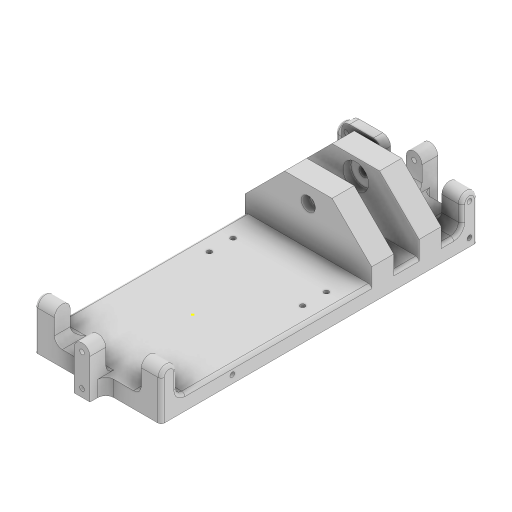
# Autodesk Inventor part: Base
Saved by Autodesk Inventor 2023 (Build 270158000, 158)
## iProperties
Created: 2023-10-18
Part Number: Base
Material: Generic
Document SubType Name: Modeling
Designer: MVeszpremi
Density: 1 g/cm^3
Appearance: Default
Author: MVeszpremi
Autodesk Inventor part; units mm, degrees
ref_plane "YZ Plane" through (0, 0, 0) normal (1, 0, 0) x (0, 1, 0)
ref_plane "XZ Plane" through (0, 0, 0) normal (0, 1, 0) x (-1, 0, 0)
ref_plane "XY Plane" through (0, 0, 0) normal (0, 0, 1) x (1, 0, 0)
sketch "Sketch1" plane through (0, 0, 0) normal (0, 1, 0) x (-1, 0, 0)
  line L0 (40, 60) -> (-40, 60)
  line L1 (-40, 60) -> (-40, -140)
  line L2 (-40, -140) -> (40, -140)
  line L3 (40, -140) -> (40, 60)
  line L4 (29.5, -40) -> (-29.5, -40)
  line L5 (-29.5, -40) -> (-29.5, -55)
  line L6 (-29.5, -55) -> (29.5, -55)
  line L7 (29.5, -55) -> (29.5, -40)
  circle A0 centre (29.5, -40) radius 1.55
  circle A1 centre (29.5, -55) radius 1.55
  circle A2 centre (-29.5, -55) radius 1.55
  circle A3 centre (-29.5, -40) radius 1.55
  point P0 (0, 0)
  dimension "d0" = 40
  dimension "d1" = 80
  dimension "d2" = 59
  dimension "d3" = 15
  dimension "d4" = 29.5
  dimension "d5" = 200
  dimension "d6" = 100
  dimension "d7" = 60
  dimension "d8" = 3.1
  dimension "d9" = 3.1
  dimension "d10" = 3.1
  dimension "d11" = 3.1
  constraints: 16 end point, 4 centre point, 4 coincident, 4 parallel, 2 horizontal, 2 perpendicular
  measures "d0" distance from line of L3 point (0, 0)
  measures "d1" distance of L0.start L0.end
  measures "d2" distance of L4.start L4.end
  measures "d3" distance of L6.end L4.start
  measures "d4" distance from line of point (0, 0) L7
  measures "d5" distance of L2.end L0.start
  measures "d6" distance between parallel lines of L0 L4
  measures "d7" distance from line of L0 point (0, 0)
  measures "d8" diameter of A0
  measures "d9" diameter of A1
  measures "d10" diameter of A3
  measures "d11" diameter of A2
extrude "Extrusion1" add sketch "Sketch1" along normal blind 10 contours L3 L2 L1 L0 | L4 A0 L7 A1 L6 A2 L5 A3
sketch "Sketch2" plane through (0, 0, 0) normal (0, -1, 0) x (1, 0, 0)
  circle A0 centre (29.5, -40) radius 1.55 projected
  line L0 (26.1802, -40) -> (27.8401, -37.125)
  line L1 (27.8401, -37.125) -> (31.1599, -37.125)
  line L2 (31.1599, -37.125) -> (32.8198, -40)
  line L3 (32.8198, -40) -> (31.1599, -42.875)
  line L4 (31.1599, -42.875) -> (27.8401, -42.875)
  line L5 (27.8401, -42.875) -> (26.1802, -40)
  circle A1 centre (29.5, -55) radius 1.55 projected
  line L6 (26.1802, -55) -> (27.8401, -52.125)
  line L7 (27.8401, -52.125) -> (31.1599, -52.125)
  line L8 (31.1599, -52.125) -> (32.8198, -55)
  line L9 (32.8198, -55) -> (31.1599, -57.875)
  line L10 (31.1599, -57.875) -> (27.8401, -57.875)
  line L11 (27.8401, -57.875) -> (26.1802, -55)
  line L12 (0, 0) -> (0, -8.5625)
  circle A2 centre (-29.5, -40) radius 1.55
  line L13 (-26.1802, -40) -> (-27.8401, -37.125)
  line L14 (-27.8401, -37.125) -> (-31.1599, -37.125)
  line L15 (-31.1599, -37.125) -> (-32.8198, -40)
  line L16 (-32.8198, -40) -> (-31.1599, -42.875)
  line L17 (-31.1599, -42.875) -> (-27.8401, -42.875)
  line L18 (-27.8401, -42.875) -> (-26.1802, -40)
  circle A3 centre (-29.5, -55) radius 1.55
  line L19 (-26.1802, -55) -> (-27.8401, -52.125)
  line L20 (-27.8401, -52.125) -> (-31.1599, -52.125)
  line L21 (-31.1599, -52.125) -> (-32.8198, -55)
  line L22 (-32.8198, -55) -> (-31.1599, -57.875)
  line L23 (-31.1599, -57.875) -> (-27.8401, -57.875)
  line L24 (-27.8401, -57.875) -> (-26.1802, -55)
  point P0 (29.5, -42.875)
  point P1 (29.5, -37.125)
  point P2 (-29.5, -42.875)
  point P3 (-29.5, -37.125)
  dimension "d14" = 5.75
  dimension "d15" = 5.75
  constraints: 50 end point, 18 symmetric about line, 4 coincident, 2 centre point, 2 midpoint, 1 vertical, 28 other
  measures "d14" distance of point (29.5, -42.875) point (29.5, -37.125)
  measures "d15" distance between parallel lines of L10 L7
extrude "Extrusion2" cut sketch "Sketch2" against normal blind 3.5 contours A0 | L0 L1 L2 L3 L4 L5 | A1 | L6 L7 L8 L9 L10 L11 | A2 | L18 L17 L16 L15 L14 L13 | A3 | L24 L23 L22 L21 L20 L19
sketch "Sketch3" plane through (0, 10, 0) normal (0, 1, 0) x (1, 0, 0)
  line L0 (-40, 140) -> (-40, -60) projected
  line L1 (40, -60) -> (40, 140) projected
  line L2 (-40, 73.125) -> (40, 73.125)
  line L3 (40, 73.125) -> (40, 87.125)
  line L4 (40, 87.125) -> (-40, 87.125)
  line L5 (-40, 87.125) -> (-40, 73.125)
  circle A0 centre (-29.5, 55) radius 1.55 projected
  line L6 (-40, 140) -> (-40, -60) projected
  line L7 (40, 103.125) -> (-40, 103.125)
  line L8 (-40, 103.125) -> (-40, 117.125)
  line L9 (-40, 117.125) -> (40, 117.125)
  line L10 (40, 117.125) -> (40, 103.125)
  point P0 (0, 0)
  point P1 (-40, 87.125)
  point P2 (40, 73.125)
  point P3 (-40, 117.125)
  point P4 (-40, 103.125)
  dimension "d18" = 18.125
  dimension "d19" = 14
  dimension "d32" = 16
  dimension "d33" = 14
  constraints: 16 end point, 4 parallel, 4 point on line, 2 horizontal, 2 perpendicular
  measures "d18" distance from line of L2 A0.centre
  measures "d19" distance between parallel lines of L4 L2
  measures "d32" distance between parallel lines of L7 L4
  measures "d33" distance between parallel lines of L9 L7
extrude "Extrusion3" add sketch "Sketch3" along normal blind 35 contours L9 L1 L7 L0 | L4 L1 L2 L0
sketch "Sketch4" plane through (40, 10, -87.125) normal (0, 0, -1) x (-1, 0, 0)
  circle A0 centre (40, 24.5) radius 8.125
  line L0 (0, 0) -> (80, 0) projected
  circle A1 centre (40, 24.5) radius 3
  point P0 (40, -10)
  point P1 (40, 0)
  dimension "d22" = 16.25
  dimension "d23" = 24.5
  dimension "d24" = 6
  constraints: 2 centre point, 1 coincident, 1 midpoint
  measures "d22" diameter of A0
  measures "d23" distance of point (40, 0) A0.centre
  measures "d24" diameter of A1
extrude "Extrusion4" cut sketch "Sketch4" along normal blind 40 and the other way blind 20 contours A1
extrude "Extrusion5" cut sketch "Sketch4" along normal blind 21 and the other way blind 5
chamfer "Chamfer1" distance 25 angle 45 4 edges at (40, 45, -80.125) (-40, 45, -80.125) (40, 45, -110.125) (-40, 45, -110.125)
sketch "Sketch5" plane through (-40, 10, -73.125) normal (0, 0, 1) x (1, 0, 0)
  circle A0 centre (40, 24.5) radius 3 projected
  circle A1 centre (40, 24.5) radius 4.5
  point P0 (40, -10)
  dimension "d38" = 9
  constraints: 1 centre point, 1 coincident
  measures "d38" diameter of A1
extrude "Extrusion6" cut sketch "Sketch5" against normal blind 5
ref_plane "Work Plane1" through (-40, 10, -110.125) normal (0, 0, 1) x (1, 0, 0)
mirror "Mirror1" about plane through (-40, 10, -110.125) normal (0, 0, 1) of "Extrusion5"
sketch "Sketch6" plane through (-40, 0, -140) normal (-1, 0, 0) x (0, 0, 1)
  point P0 (140, 0)
sketch "Sketch7" plane through (-40, 0, -140) normal (-1, 0, 0) x (0, 0, 1)
  line L0 (0, 0) -> (0, 10) projected
  line L1 (0, 10) -> (10, 10)
  line L2 (10, 10) -> (10, 30)
  line L3 (10, 30) -> (0, 30)
  line L4 (0, 30) -> (0, 10)
  line L5 (200, 10) -> (66.875, 10) projected
  line L6 (200, 10) -> (190, 10)
  line L7 (190, 10) -> (190, 30)
  line L8 (190, 30) -> (200, 30)
  line L9 (200, 30) -> (200, 10)
  circle A0 centre (5, 25) radius 1.5
  circle A1 centre (155, 25) radius 1.5
  point P0 (140, 0)
  point P1 (190, 10)
  dimension "d41" = 150
  dimension "d42" = 5
  dimension "d43" = 20
  dimension "d44" = 10
  dimension "d45" = 3
  dimension "d46" = 10
  dimension "d47" = 20
  dimension "d48" = 3
  dimension "d51" = 15
  dimension "d52" = 15
  constraints: 16 end point, 4 parallel, 2 centre point, 2 horizontal, 2 perpendicular
  measures "d41" distance of A1.centre A0.centre
  measures "d42" distance from line of L0 A0.centre
  measures "d43" distance of L6.end L7.end
  measures "d44" distance of L7.end L8.end
  measures "d45" diameter of A1
  measures "d46" distance of L2.end L3.end
  measures "d47" distance of L1.end L2.end
  measures "d48" diameter of A0
  measures "d51" distance from line of L5 A1.centre
  measures "d52" distance from line of L1 A0.centre
extrude "Extrusion7" add sketch "Sketch7" against normal blind 12.5 contours L4 L3 L2 L1 | L5 L7 L8 L9
ref_plane "Work Plane2" through (0, 0, -140) normal (-1, 0, 0) x (0, 0, 1)
mirror "Mirror2" about plane through (0, 0, -140) normal (-1, 0, 0) of "Extrusion7"
sketch "Sketch8" plane through (-40, 0, -140) normal (-1, 0, 0) x (0, 0, 1)
  circle A0 centre (5, 5) radius 1.5
  circle A1 centre (155, 5) radius 1.5
  line L0 (0, 0) -> (0, 30) projected
  line L1 (0, 0) -> (200, 0) projected
  point P0 (140, 0)
  dimension "d53" = 150
  dimension "d54" = 5
  dimension "d55" = 5
  dimension "d56" = 3
  dimension "d57" = 3
  constraints: 2 centre point, 1 horizontal alignment
  measures "d53" distance of A1.centre A0.centre
  measures "d54" distance from line of L0 A0.centre
  measures "d55" distance from line of L1 A0.centre
  measures "d56" diameter of A0
  measures "d57" diameter of A1
extrude "Extrusion8" cut sketch "Sketch8" against normal blind 15
mirror "Mirror3" about plane through (0, 0, -140) normal (-1, 0, 0) of "Extrusion8"
sketch "Sketch9" plane through (-40, 0, 60) normal (0, 0, 1) x (1, 0, 0)
  line L0 (0, 0) -> (80, 0) projected
  line L1 (35, 0) -> (45, 0)
  line L2 (45, 0) -> (45, 30)
  line L3 (45, 30) -> (35, 30)
  line L4 (35, 30) -> (35, 0)
  circle A0 centre (40, 25) radius 1.5
  circle A1 centre (40, 5) radius 1.5
  point P0 (40, 0)
  point P1 (40, 0)
  point P2 (40, 0)
  point P3 (40, 0)
  dimension "d60" = 5
  dimension "d61" = 5
  dimension "d62" = 30
  dimension "d63" = 5
  dimension "d64" = 20
  dimension "d65" = 3
  dimension "d66" = 3
  constraints: 8 end point, 3 midpoint, 2 centre point, 2 parallel, 1 horizontal, 1 perpendicular, 1 point on line
  measures "d60" distance from line of L4 point (40, 0)
  measures "d61" distance from line of point (40, 0) L2
  measures "d62" distance of L1.end L2.end
  measures "d63" distance of point (40, 0) A1.centre
  measures "d64" distance of A1.centre A0.centre
  measures "d65" diameter of A0
  measures "d66" diameter of A1
extrude "Extrusion9" add sketch "Sketch9" along normal blind 10
ref_plane "Work Plane3" through (40, 0, -40) normal (0, 0, -1) x (-1, 0, 0)
mirror "Mirror4" about plane through (40, 0, -40) normal (0, 0, -1) of "Extrusion9"
fillet "Fillet1" radius 5 26 edges at (5, 5, 60) (-5, 5, 60) (-5, 30, 65) (5, 30, 65) (-33.75, 30, 60) (-33.75, 30, 50) (33.75, 30, 60) (33.75, 30, 50) (27.5, 10, 55) (-27.5, 10, 55) (33.75, 10, 50) (-33.75, 10, 50) (33.75, 30, -140) (33.75, 30, -130) (33.75, 10, -130) (5, 30, -145) (-5, 30, -145) (0, 10, -140) (0, 10, 60) (-5, 5, -140) (5, 5, -140) (-27.5, 10, -135) (-33.75, 30, -140) (-33.75, 30, -130) (-33.75, 10, -130) (27.5, 10, -135)
fillet "Fillet2" radius 2 22 edges at (-40, 11.4645, 48.5355) (-40, 20, 50) (-40, 30, 55) (-40, 12.5, 60) (-40, 10, -14.0625) (-40, 10, -95.125) (-40, 11.4645, -128.5355) (-40, 20, -130) (-40, 30, -135) (-40, 12.5, -140) (-40, 10, -121.0625) (40, 11.4645, 48.5355) (40, 20, 50) (40, 30, 55) (40, 12.5, 60) (40, 10, -14.0625) (40, 10, -95.125) (40, 11.4645, -128.5355) (40, 20, -130) (40, 30, -135) (40, 12.5, -140) (40, 10, -121.0625)
sketch "Sketch10" plane through (0, 10, 0) normal (0, 1, 0) x (1, 0, 0)
  point P0 (0, 0)
sketch "Sketch11" plane through (0, 10, 0) normal (0, 1, 0) x (1, 0, 0)
  line L0 (-5, 124.125) -> (-30, 124.125)
  line L1 (-30, 124.125) -> (-30, 130.125)
  line L2 (-30, 130.125) -> (-5, 130.125)
  line L3 (-5, 130.125) -> (-5, 124.125)
  line L4 (15, 117.125) -> (-15, 117.125) projected
  point P0 (0, 0)
  dimension "d71" = 5
  dimension "d72" = 25
  dimension "d73" = 6
  dimension "d76" = 7
  constraints: 8 end point, 2 parallel, 1 horizontal, 1 perpendicular
  measures "d71" horizontal distance of L2.end point (0, 0)
  measures "d72" distance of L0.start L0.end
  measures "d73" distance of L0.end L1.end
  measures "d76" distance between parallel lines of L4 L0
extrude "Extrusion10" add sketch "Sketch11" along normal blind 30
sketch "Sketch12" plane through (-5, 10, -130.125) normal (0, 0, -1) x (-1, 0, 0)
  circle A0 centre (3, 24.5) radius 1.5
  circle A1 centre (22, 24.5) radius 1.5
  line L0 (0, 30) -> (25, 30) projected
  line L1 (12.5, 30) -> (12.5, 24.5)
  circle A2 centre (-5, 24.5) radius 3 projected
  line L2 (8.5, 28) -> (16.5, 28)
  line L3 (16.5, 28) -> (16.5, 21)
  line L4 (16.5, 21) -> (8.5, 21)
  line L5 (8.5, 21) -> (8.5, 28)
  point P0 (-5, -10)
  point P1 (12.5, 27.25)
  dimension "d77" = 3
  dimension "d78" = 3
  dimension "d79" = 9.5
  dimension "d80" = 9.5
  dimension "d81" = 7
  dimension "d82" = 2
  dimension "d83" = 8
  dimension "d84" = 4
  constraints: 10 end point, 2 centre point, 2 horizontal alignment, 2 midpoint, 2 parallel, 1 horizontal, 1 perpendicular, 1 vertical
  measures "d77" diameter of A0
  measures "d78" diameter of A1
  measures "d79" distance from line of L1 A0.centre
  measures "d80" distance from line of A1.centre L1
  measures "d81" distance of L4.end L2.start
  measures "d82" distance between parallel lines of L0 L2
  measures "d83" distance of L2.start L2.end
  measures "d84" distance from line of point (12.5, 27.25) L5
extrude "Extrusion11" cut sketch "Sketch12" against normal blind 6 contours A0 | A1
extrude "Extrusion12" cut sketch "Sketch12" against normal blind 4 contours L2 L3 L4 L5
fillet "Fillet3" radius 5 2 edges at (-5, 40, -127.125) (-30, 40, -127.125)
body "Solid1"
